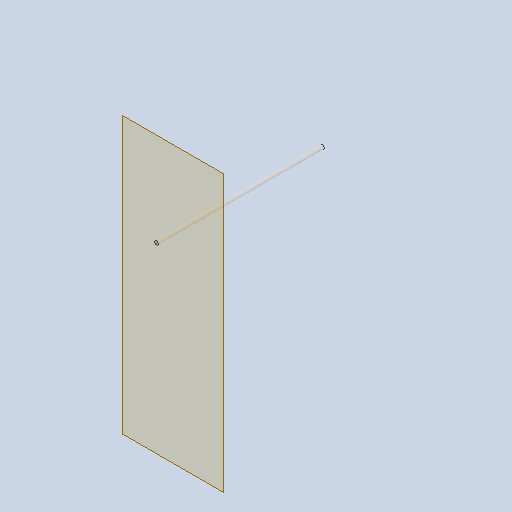
# Autodesk Inventor part: спиралька
Saved by Autodesk Inventor 2024.2 (Build 282272000, 272)
## iProperties
Created: 2026-02-10
Part Number: спиралька
Material: Типовые
Document SubType Name: Modeling
Designer: Service
Density: 1 g/cm^3
Appearance: По умолчанию
Author: Service
Autodesk Inventor part; units mm, degrees
ref_plane "YZ Plane" through (0, 0, 0) normal (1, 0, 0) x (0, 1, 0)
ref_plane "XZ Plane" through (0, 0, 0) normal (0, 1, 0) x (-1, 0, 0)
ref_plane "XY Plane" through (0, 0, 0) normal (0, 0, 1) x (1, 0, 0)
ref_plane "РабПлоскость1" through (0, 62.5862, 0) normal (0, 0, 1) x (1, 0, 0)
sketch "Эскиз1" plane through (0, 62.5862, 0) normal (0, 0, 1) x (1, 0, 0)
  circle A0 centre (-18, 69.4138) radius 7 projected
  circle A1 centre (-18, 69.4138) radius 2
  point P0 (0, -62.5862)
  dimension "d0" = 4
  constraints: 1 centre point, 1 coincident
  measures "d0" diameter of A1
extrude "Выдавливание1" add sketch "Эскиз1" against normal blind 180 contours A1
